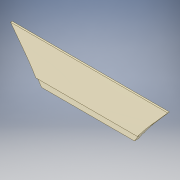
# Autodesk Inventor part: bachi_v2
Saved by Autodesk Inventor 2019 (Build 230136000, 136)
## iProperties
Created: 2020-11-22
Part Number: bachi_v2
Material: Фарфор, слоновая кость
Document SubType Name: Modeling
Designer: stepa
Density: 3.4 g/cm^3
Appearance: Солнечный день
Mass: 14.6209 g
Surface Area: 40.6615 cm^2
Volume: 4.30026 cm^3
Author: stepa
Autodesk Inventor part; units mm, degrees
ref_plane "YZ Plane" through (0, 0, 0) normal (1, 0, 0) x (0, 1, 0)
ref_plane "XZ Plane" through (0, 0, 0) normal (0, 1, 0) x (-1, 0, 0)
ref_plane "XY Plane" through (0, 0, 0) normal (0, 0, 1) x (1, 0, 0)
sketch "Эскиз1" plane through (0, 0, 0) normal (0, 0, 1) x (1, 0, 0)
  line L0 (-13, 0) -> (13, 0)
  line L1 (-47.5, 180) -> (47.5, 180)
  line L2 (-16.5, 130) -> (16.5, 130)
  line L3 (-12.9827, 110) -> (12.9827, 110)
  line L4 (-11.8003, 90) -> (11.8003, 90)
  line L5 (47.5, 180) -> (37.594, 168.7363)
  line L6 (-47.5, 180) -> (-37.594, 168.7363)
  line L7 (-37.594, 168.7363) -> (37.594, 168.7363)
  arc A0 (37.594, 168.7363) -> (12.9827, 110) centre (112.573, 102.7948) ccw
  arc A1 (12.9827, 110) -> (13, 0) centre (771.5375, 55.1194) ccw
  arc A2 (-12.9827, 110) -> (-37.594, 168.7363) centre (-112.573, 102.7948) ccw
  arc A3 (-13, 0) -> (-12.9827, 110) centre (-771.5375, 55.1194) ccw
  line L8 (-11, 80.4723) -> (-11, 26.1046)
  line L9 (11, 80.4723) -> (11, 26.1046)
  line L10 (-37.594, 168.7363) -> (13.0707, 111.1279)
  line L11 (37.594, 168.7363) -> (-13.0707, 111.1279)
  point P0 (0, 0)
  point P1 (0, 0)
  point P2 (0, 180)
  point P3 (0, 130)
  point P4 (0, 90)
  point P5 (0, 110)
  point P6 (-11, 55.1194)
  dimension "d0" = 26
  dimension "d1" = 95
  dimension "d2" = 33
  dimension "d5" = 180
  dimension "d6" = 50
  dimension "d7" = 20
  dimension "d8" = 20
  dimension "d9" = 15
  dimension "d10" = 15
  dimension "d13" = 22
  dimension "d19" = 55.1194
  constraints: 24 end point, 15 point on circle, 6 horizontal, 5 midpoint, 4 centre point, 4 tangent, 4 vertical alignment, 2 coincident, 2 collinear, 2 vertical, 1 horizontal alignment, 1 point on line
  measures "d0" distance of L0.start L0.end
  measures "d1" distance of L1.start L1.end
  measures "d2" distance of L2.start L2.end
  measures "d5" distance between parallel lines of L1 L0
  measures "d6" distance between parallel lines of L1 L2
  measures "d7" distance between parallel lines of L3 L2
  measures "d8" distance between parallel lines of L3 L4
  measures "d9" distance of L1.end L5.end
  measures "d10" distance of L1.start L6.end
  measures "d13" distance between parallel lines of L9 L8
  measures "d19" distance from line of L0 point (-11, 55.119)
extrude "Выдавливание1" add sketch "Эскиз1" along normal blind 25
sketch "Эскиз2" plane through (0, 0, 0) normal (1, 0, 0) x (0, 1, 0)
  line L0 (0, 0) -> (110, 0) projected
  line L1 (110, 0) -> (110, 25) projected
  line L2 (0, 25) -> (110, 25) projected
  line L3 (0, 0) -> (0, 25) projected
  line L4 (110, 0) -> (169.3956, 0) projected
  line L5 (110, 25) -> (169.3956, 25) projected
  line L6 (110, 0) -> (110, 25) projected
  line L7 (130, 18) -> (130, 7)
  line L8 (55, 21) -> (55, 4)
  arc A0 (0, 25) -> (130, 18) centre (172.2556, 2013.3889) ccw
  arc A1 (130, 7) -> (0, 0) centre (172.2556, -1988.3889) ccw
  line L9 (180, 13) -> (180, 12)
  line L10 (160, 14.5) -> (160, 10.5)
  line L11 (180, 13) -> (160, 14.5)
  line L12 (180, 12) -> (160, 10.5)
  arc A2 (130, 18) -> (160, 14.5) centre (187.3675, 379.4) ccw
  arc A3 (160, 10.5) -> (130, 7) centre (187.3675, -354.4) ccw
  line L13 (168.7363, 0) -> (180, 0) projected
  line L14 (180, 0) -> (180, 25) projected
  line L15 (168.7363, 25) -> (180, 25) projected
  line L16 (160, 13.75) -> (156, 13.75)
  line L17 (156, 13.75) -> (156, 11.25)
  line L18 (156, 11.25) -> (160, 11.25)
  point P0 (130, 12.5)
  point P1 (0, 12.5)
  point P2 (55, 12.5)
  point P3 (180, 12.5)
  point P4 (169.3956, 12.5)
  point P5 (160, 12.5)
  point P6 (180, 12.5)
  point P7 (156, 12.5)
  dimension "d16" = 11
  dimension "d20" = 55
  dimension "d21" = 17
  dimension "d22" = 1
  dimension "d23" = 4
  dimension "d28" = 50
  dimension "d30" = 20
  dimension "d33" = 4
  dimension "d34" = 2.5
  constraints: 18 end point, 10 point on circle, 7 midpoint, 4 centre point, 4 horizontal alignment, 4 vertical, 2 coincident, 2 perpendicular, 2 point on line, 2 tangent, 1 equal length, 1 horizontal
  measures "d16" distance of L7.start L7.end
  measures "d20" distance between parallel lines of L3 L8
  measures "d21" distance of L8.start L8.end
  measures "d22" distance of L9.start L9.end
  measures "d23" distance of L10.start L10.end
  measures "d28" distance between parallel lines of L14 L7
  measures "d30" distance between parallel lines of L10 L9
  measures "d33" distance of L17.end L18.end
  measures "d34" distance of L16.end L17.end
extrude "Выдавливание2" cut sketch "Эскиз2" along normal mid plane 100 contours L10 L11 L9 L12 | L18 L17 L16 L10 keep common part
